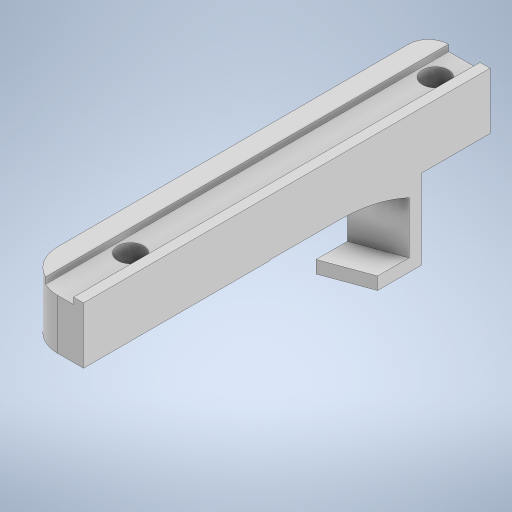
# Autodesk Inventor part: Right-Brush-Bottom
Saved by Autodesk Inventor 2024 (Build 280153000, 153)
## iProperties
Created: 2023-12-12
Part Number: Right-Brush-Bottom
Material: Generic
Document SubType Name: Modeling
Designer: shaun
Density: 1 g/cm^3
Appearance: Default
Author: shaun
Autodesk Inventor part; units mm, degrees
ref_plane "YZ Plane" through (0, 0, 0) normal (1, 0, 0) x (0, 1, 0)
sketch "Sketch1" plane through (0, 0, 0) normal (0, 1, 0) x (-1, 0, 0)
  line L0 (0, 0) -> (11.4, 0) construction
  line L1 (11.4, 0) -> (11.4, -64.7) construction
  line L2 (11.4, -64.7) -> (0, -64.7) construction
  line L3 (0, -64.7) -> (0, 0) construction
  line L4 (5.7, 0) -> (5.7, -64.7) construction
  line L5 (11.4, -32.35) -> (0, -32.35) construction
  circle A0 centre (5.7, -11.6) radius 1.6 construction
  circle A1 centre (5.7, -11.6) radius 2.05
  circle A2 centre (5.7, -21.3) radius 1.6 construction
  circle A3 centre (5.7, -21.3) radius 2.05 construction
  circle A4 centre (5.7, -31) radius 1.6 construction
  circle A5 centre (5.7, -31) radius 2.05 construction
  circle A6 centre (5.7, -40.7) radius 1.6 construction
  circle A7 centre (5.7, -40.7) radius 2.05 construction
  circle A8 centre (5.7, -50.4) radius 1.6 construction
  circle A9 centre (5.7, -50.4) radius 2.05 construction
  circle A10 centre (5.7, -60.1) radius 1.6 construction
  circle A11 centre (5.7, -60.1) radius 2.05
  line L6 (8.2, 0) -> (3.2, 0) construction
  line L7 (3.2, 0) -> (3.2, -64.7)
  line L8 (3.2, -64.7) -> (8.2, -64.7) construction
  line L9 (8.2, -64.7) -> (8.2, 0)
  circle A12 centre (5.7, -11.6) radius 2.5 construction
  circle A13 centre (5.7, -5.7) radius 5.7 construction
  circle A14 centre (8.2, -61.5) radius 3.2 construction
  line L10 (0, -64.7) -> (3.2, -64.7) construction
  line L11 (1.6, -64.7) -> (1.6, 0)
  circle A15 centre (5.7, -60.1) radius 3.65
  circle A16 centre (5.7, -50.4) radius 3.65 construction
  circle A17 centre (5.7, -40.7) radius 3.65 construction
  circle A18 centre (5.7, -31) radius 3.65 construction
  circle A19 centre (5.7, -21.3) radius 3.65 construction
  circle A20 centre (5.7, -11.6) radius 3.65
  arc A21 (8.2, -64.7) -> (11.4, -61.5) centre (8.2, -61.5) ccw
  arc A22 (11.4, -5.7) -> (5.7, 0) centre (5.7, -5.7) ccw
  line L12 (11.4, -61.5) -> (11.4, -5.7)
  line L13 (1.6, -64.7) -> (8.2, -64.7)
  line L14 (1.6, 0) -> (5.7, 0)
  point P0 (5.7, -10)
  point P1 (5.7, -61.7)
  point P2 (8.2, -0.5775)
  dimension "d0" = 3.2
  dimension "d1" = 4.1
  dimension "d4" = 9.7
  dimension "d9" = 6.5
  dimension "d10" = 10
  dimension "d11" = 3
  dimension "d12" = 0.9
  dimension "d13" = 3.2
  dimension "d14" = 7.3
  dimension "d39" = 48.5
  constraints: 30 end point, 21 centre point, 16 coincident, 10 point on line, 8 point on circle, 5 equal radius, 5 midpoint, 5 parallel, 5 tangent, 3 perpendicular, 2 collinear, 2 horizontal, 2 line through centre, 2 vertical, 2 vertical alignment, 22 other
  measures "d1" diameter of A1
  measures "d4" distance of point (5.7, -11.6) A2.centre
  measures "d10" distance from line of L0 point (5.7, -10)
  measures "d11" distance of L4.end point (5.7, -61.7)
  measures "d13" distance between parallel lines of L1 L9
  measures "d14" diameter of A15
  measures "d39" distance of A20.centre A15.centre
extrude "Extrusion1" add sketch "Sketch1" along normal blind 6 contours L7 A20 A15 L13 L11 L14 | L7 A20 | A20 L9 | L9 A22 L12 A21 A15 A20 | L7 A15 | A15 L9
extrude "Extrusion3" add sketch "Sketch1" along normal blind 5 contours L14 A22 L9 A20 L7 | A20 L9 L7 | A20 L9 A15 L7 | A15 L9 L7 | L7 A15 L9 L13
extrude "Extrusion2" add sketch "Sketch1" against normal blind 3 contours L14 A22 L9 A20 L7 | L7 A20 A15 L13 L11 L14 | A20 L9 A15 L7 | L9 A22 L12 A21 A15 A20 | L7 A15 L9 L13
sketch "Sketch2" plane through (0, -3, 0) normal (0, -1, 0) x (1, 0, 0)
  line L0 (-1.6, -64.7) -> (-1.6, 0) construction
  circle A0 centre (-5.7, -11.6) radius 3.65 construction
  circle A1 centre (-5.7, -60.1) radius 3.65 construction
  line L1 (-11.4, -5.7) -> (-11.4, -61.5) construction
  arc A2 (-11.4, -61.5) -> (-8.2, -64.7) centre (-8.2, -61.5) ccw construction
  line L2 (-8.2, -64.7) -> (-1.6, -64.7) construction
  arc A3 (-5.7, 0) -> (-11.4, -5.7) centre (-5.7, -5.7) ccw construction
  line L3 (-1.6, 0) -> (-5.7, 0) construction
  line L4 (-5.7, -60.1) -> (-5.7, -11.6) construction
  circle A4 centre (-5.7, -55.25) radius 4.85 construction
  circle A5 centre (-5.7, -45.55) radius 4.85 construction
  circle A6 centre (-5.7, -35.85) radius 4.85 construction
  circle A7 centre (-5.7, -26.15) radius 4.85 construction
  circle A8 centre (-5.7, -16.45) radius 4.85 construction
  line L5 (0, -51.8) -> (-11.4, -51.8) construction
  line L6 (-11.4, -51.8) -> (-11.4, -29.6) construction
  line L7 (-11.4, -29.6) -> (0, -29.6) construction
  line L8 (0, -29.6) -> (0, -51.8) construction
  line L9 (0, -51.8) -> (-11.4, -29.6) construction
  line L10 (-11.4, -51.8) -> (0, -29.6) construction
  line L11 (0, -27.1) -> (-11.4, -27.1) construction
  line L12 (-11.4, -27.1) -> (-11.4, -54.3) construction
  line L13 (-11.4, -54.3) -> (0, -54.3) construction
  line L14 (0, -54.3) -> (0, -27.1) construction
  line L15 (0, -27.1) -> (-11.4, -54.3) construction
  line L16 (-11.4, -27.1) -> (0, -54.3) construction
  line L17 (-11.4, -54.3) -> (-1.6, -54.3)
  line L18 (-1.6, -54.3) -> (-1.6, -51.8)
  line L19 (-1.6, -51.8) -> (-11.4, -51.8)
  line L20 (-11.4, -51.8) -> (-11.4, -54.3)
  point P0 (0, 0)
  point P1 (-5.7, -50.4)
  point P2 (-5.7, -40.7)
  point P3 (-5.7, -31)
  point P4 (-5.7, -21.3)
  dimension "d21" = 22.2
  dimension "d22" = 2.5
  constraints: 32 end point, 10 point on circle, 6 parallel, 5 centre point, 4 equal radius, 4 midpoint, 4 point on line, 3 horizontal, 3 perpendicular, 12 other
  measures "d21" distance of L5.end L6.end
  measures "d22" distance between parallel lines of L5 L13
ref_plane "Work Plane1" through (-1.6, -3, -51.8) normal (0, 0, 1) x (1, 0, 0)
sketch "Sketch3" plane through (-1.6, -3, -51.8) normal (0, 0, 1) x (1, 0, 0)
  line L0 (0, 0) -> (-9.8, 0) projected
  line L1 (0, 0) -> (0, -2.4)
  line L2 (0, -2.4) -> (-9.8, -5.0259)
  line L3 (-9.8, -5.0259) -> (-9.8, 0)
  line L4 (0, -2.4) -> (-9.8, -2.4) construction
  line L5 (0, -2.4) -> (0, -10.6822)
  line L6 (0, -10.6822) -> (-9.8, -13.3081)
  line L7 (-9.8, -13.3081) -> (-9.8, -5.0259)
  line L8 (-9.8, -13.3081) -> (-9.8, -15.3081)
  line L9 (-9.8, -15.3081) -> (0, -12.6822)
  line L10 (0, -12.6822) -> (0, -10.6822)
  line L11 (-9.8, -5.0259) -> (-7.7294, -12.7533) construction
  point P0 (1.6, 3)
  dimension "d23" = 2.4
  dimension "d24" = 15
  dimension "d25" = 9.8
  dimension "d26" = 2
  dimension "d27" = 8
  constraints: 22 end point, 4 parallel, 4 point on line, 3 perpendicular, 2 vertical
  measures "d23" distance of L0.start L1.end
  measures "d24" angle of L4 L2
  measures "d25" distance of L1.end L4.end
  measures "d26" distance of L8.end L6.end
  measures "d27" distance of L2.end L11.end
extrude "Extrusion4" add sketch "Sketch3" against normal blind 2
extrude "Extrusion5" add sketch "Sketch3" along normal blind 22.2 contours L1 L2 L3 L0
ref_plane "Work Plane2" through (-11.4, -8.0259, -51.8) normal (-0.9659, -0.2588, 0) x (0.2588, -0.9659, 0)
sketch "Sketch4" plane through (-11.4, -8.0259, -51.8) normal (-0.9659, -0.2588, 0) x (0.2588, -0.9659, 0)
  line L0 (0, 0) -> (0, 22.2) projected
  arc A0 (0, 22.2) -> (0, 0) centre (24.4688, 11.1) ccw
  line L1 (-2.4, 11.1) -> (-2.4273, 22.2)
  line L2 (-4.8546, 22.2) -> (0, 22.2) projected
  line L3 (0, 22.2) -> (-2.4273, 22.2)
  point P0 (-4.8019, 51.8)
  point P1 (0, 11.1)
  dimension "d32" = 2.4
  constraints: 4 end point, 3 point on circle, 2 midpoint, 1 centre point
  measures "d32" distance of L1.start point (0, 11.1)
extrude "Extrusion6" cut sketch "Sketch4" against normal through all
extrude "Extrusion7" add sketch "Sketch3" along normal blind 5 contours L10 L9 L8 L6
body "Solid1"
